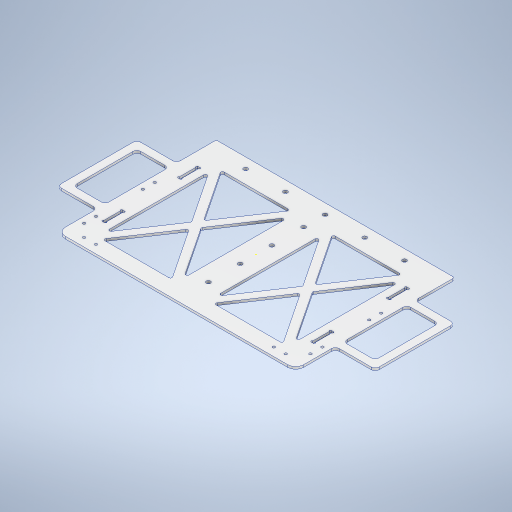
# Autodesk Inventor part: RP_Waist-Avobe-ver2
Saved by Autodesk Inventor 2024.3 (Build 283343000, 343)
## iProperties
Created: 2025-04-20
Part Number: RP_Waist-Avobe-ver2
Material: アルミニウム 6061
Document SubType Name: Modeling
Designer: ngt-a
Density: 2.7 g/cm^3
Appearance: アルミニウム - フラット
Mass: 310.216 g
Surface Area: 892.206 cm^2
Volume: 114.895 cm^3
Author: ngt-a
Autodesk Inventor part; units mm, degrees
ref_plane "YZ Plane" through (0, 0, 0) normal (1, 0, 0) x (0, 1, 0)
ref_plane "XZ Plane" through (0, 0, 0) normal (0, 1, 0) x (-1, 0, 0)
ref_plane "XY Plane" through (0, 0, 0) normal (0, 0, 1) x (1, 0, 0)
sketch "スケッチ1" plane through (0, 0, 0) normal (0, 1, 0) x (-1, 0, 0)
  line L0 (150, -95) -> (-150, -95)
  line L1 (-150, -95) -> (-150, 95)
  line L2 (-150, 95) -> (150, 95)
  line L3 (150, 95) -> (150, -95)
  line L4 (150, -95) -> (-150, 95) construction
  line L5 (-150, -95) -> (150, 95) construction
  line L6 (150, 95) -> (-150, 95)
  line L7 (-150, 95) -> (-150, 100)
  line L8 (-150, 100) -> (150, 100)
  line L9 (150, 100) -> (150, 95)
  line L10 (150, -50) -> (200, -50)
  line L11 (200, -50) -> (200, 50)
  line L12 (200, 50) -> (150, 50)
  line L13 (150, 50) -> (150, -50)
  line L14 (-150, -50) -> (-200, -50)
  line L15 (-200, -50) -> (-200, 50)
  line L16 (-200, 50) -> (-150, 50)
  line L17 (-150, 50) -> (-150, -50)
  line L18 (190, -40) -> (160, -40)
  line L19 (160, -40) -> (160, 40)
  line L20 (160, 40) -> (190, 40)
  line L21 (190, 40) -> (190, -40)
  line L22 (-190, -40) -> (-160, -40)
  line L23 (-160, -40) -> (-160, 40)
  line L24 (-160, 40) -> (-190, 40)
  line L25 (-190, 40) -> (-190, -40)
  line L26 (160, -40) -> (150, -40)
  line L27 (150, -40) -> (150, 40)
  line L28 (150, 40) -> (160, 40)
  line L29 (160, 40) -> (160, -40)
  line L30 (-160, -40) -> (-150, -40)
  line L31 (-150, -40) -> (-150, 40)
  line L32 (-150, 40) -> (-160, 40)
  line L33 (-160, 40) -> (-160, -40)
  point P0 (0, 0)
  point P1 (150, 0)
  point P2 (175, -40)
  point P3 (-155, -40)
  point P4 (-155, 40)
  point P5 (-150, 40)
  point P6 (150, 40)
  dimension "d0" = 190
  dimension "d1" = 300
  dimension "d244" = 5
  dimension "d346" = 50
  dimension "d347" = 50
  dimension "d348" = 50
  dimension "d349" = 50
  dimension "d350" = 10
  dimension "d351" = 10
  dimension "d352" = 80
  constraints: 68 end point, 16 parallel, 8 perpendicular, 6 horizontal, 6 midpoint, 6 point on line, 6 other
  measures "d0" distance of L0.end L1.end
  measures "d1" distance of L0.start L0.end
  measures "d244" distance between parallel lines of L2 L8
  measures "d346" distance between parallel lines of L13 L11
  measures "d347" distance from line of point (0, 0) L10
  measures "d348" distance from line of L12 point (150, 0)
  measures "d349" distance between parallel lines of L17 L15
  measures "d350" distance from line of L10 point (175, -40)
  measures "d351" distance between parallel lines of L14 L22
  measures "d352" distance of point (-155, -40) point (-155, 40)
extrude "押し出し1" add sketch "スケッチ1" along normal blind 3 contours L0 L1 L2 L3 | L3 L26 L18 L21 L20 L28 L12 L11 L10 | L14 L15 L16 L1 L32 L24 L25 L22 L30 | L2 L7 L8 L9
sketch "スケッチ2" plane through (0, 3, 0) normal (0, 1, 0) x (1, 0, 0)
  circle A0 centre (-142.5, -74) radius 1.6
  circle A1 centre (142.5, -74) radius 1.6
  line L0 (-150, -95) -> (150, -95) projected
  circle A2 centre (-142.5, -59) radius 1.6
  circle A3 centre (142.5, -59) radius 1.6
  circle A4 centre (-127, -89.5) radius 1.6
  line L1 (-150, 95) -> (-150, -100) projected
  circle A5 centre (-112, -89.5) radius 1.6
  line L2 (150, 95) -> (-150, 95) projected
  line L3 (0, 95) -> (0, -95)
  line L4 (-150, -2.5) -> (150, 0)
  line L5 (150, -95) -> (150, 95) projected
  circle A6 centre (127, -89.5) radius 1.6
  circle A7 centre (112, -89.5) radius 1.6
  circle A8 centre (-142.5, 15) radius 1.6
  circle A9 centre (-142.5, 0) radius 1.6
  circle A10 centre (142.5, 15) radius 1.6
  circle A11 centre (142.5, 0) radius 1.6
  point P0 (0, 0)
  dimension "d55" = 142.5
  dimension "d56" = 285
  dimension "d57" = 3.2
  dimension "d58" = 3.2
  dimension "d59" = 21
  dimension "d60" = 21
  dimension "d61" = 15
  dimension "d62" = 15
  dimension "d63" = 3.2
  dimension "d64" = 3.2
  dimension "d67" = 5.5
  dimension "d68" = 23
  dimension "d69" = 15
  dimension "d70" = 3.2
  dimension "d71" = 3.2
  dimension "d72" = 80
  dimension "d73" = 7.5
  dimension "d74" = 15
  dimension "d75" = 3.2
  dimension "d76" = 3.2
  dimension "d245" = 3.2
  constraints: 12 centre point, 4 end point, 4 midpoint, 4 symmetric about line, 4 other
  measures "d55" horizontal distance of A0.centre point (0, 0)
  measures "d56" distance of A1.centre A0.centre
  measures "d57" diameter of A0
  measures "d58" diameter of A1
  measures "d59" distance from line of L0 A0.centre
  measures "d60" distance from line of L0 A1.centre
  measures "d61" distance of A0.centre A2.centre
  measures "d62" distance of A1.centre A3.centre
  measures "d63" diameter of A3
  measures "d64" diameter of A2
  measures "d67" distance from line of L0 A4.centre
  measures "d68" distance from line of A4.centre L1
  measures "d69" distance of A5.centre A4.centre
  measures "d70" diameter of A5
  measures "d71" diameter of A4
  measures "d72" distance from line of A8.centre L2
  measures "d73" distance from line of A8.centre L1
  measures "d74" distance of A9.centre A8.centre
  measures "d75" diameter of A9
  measures "d76" diameter of A8
  measures "d245" diameter of A7
extrude "押し出し4" cut sketch "スケッチ2" against normal blind 10 contours A0 | A1 | A11 L4 | L4 A11 | A2 | A3 | A4 | A5 | A6 | A7 | A8 | A9 | A10
sketch "スケッチ4" plane through (0, 3, 0) normal (0, 1, 0) x (1, 0, 0)
  point P0 (0, 0)
sketch "スケッチ14" plane through (150, 0, -95) normal (0, 0, -1) x (-1, 0, 0)
  line L0 (0, 0) -> (300, 0) projected
  line L1 (300, 0) -> (300, 3) projected
  line L2 (0, 3) -> (300, 3) projected
  line L3 (0, 0) -> (0, 3) projected
  point P0 (150, 0)
extrude "押し出し13" add sketch "スケッチ14" along normal blind 5
fillet "フィレット3" radius 10 2 edges at (150, 1.5, 100) (-150, 1.5, 100)
sketch "スケッチ19" plane through (0, 0, 0) normal (0, -1, 0) x (1, 0, 0)
  circle A0 centre (-142.5, -15) radius 1.6 projected
  circle A1 centre (127, 89.5) radius 1.6 projected
  circle A2 centre (142.5, 74) radius 1.6 projected
  circle A3 centre (-142.5, 59) radius 1.6 projected
  circle A4 centre (-112, 89.5) radius 1.6 projected
  circle A5 centre (142.5, 0) radius 1.6 projected
  circle A6 centre (-142.5, 0) radius 1.6 projected
  circle A7 centre (112, 89.5) radius 1.6 projected
  circle A8 centre (142.5, 59) radius 1.6 projected
  circle A9 centre (-142.5, 74) radius 1.6 projected
  circle A10 centre (-127, 89.5) radius 1.6 projected
  circle A11 centre (142.5, -15) radius 1.6 projected
  line L0 (150, -40) -> (190, -40) projected
  line L1 (150, 40) -> (150, -40) projected
  line L2 (190, 40) -> (150, 40) projected
  line L3 (190, -40) -> (190, 40) projected
  line L4 (-150, 40) -> (-190, 40) projected
  line L5 (-150, -40) -> (-150, 40) projected
  line L6 (-190, -40) -> (-150, -40) projected
  line L7 (-190, 40) -> (-190, -40) projected
  arc A12 (-140, 100) -> (-150, 90) centre (-140, 90) ccw projected
  line L8 (-150, 50) -> (-150, 90) projected
  line L9 (-200, 50) -> (-150, 50) projected
  line L10 (-200, -50) -> (-200, 50) projected
  line L11 (-150, -50) -> (-200, -50) projected
  line L12 (-150, -50) -> (-150, -100) projected
  line L13 (150, -100) -> (-150, -100) projected
  line L14 (150, -50) -> (150, -100) projected
  line L15 (200, -50) -> (150, -50) projected
  line L16 (200, 50) -> (200, -50) projected
  line L17 (150, 50) -> (200, 50) projected
  line L18 (150, 90) -> (150, 50) projected
  arc A13 (150, 90) -> (140, 100) centre (140, 90) ccw projected
  line L19 (-140, 100) -> (140, 100) projected
  line L20 (120, -70) -> (20, -70)
  line L21 (20, -70) -> (20, 80)
  line L22 (20, 80) -> (120, 80)
  line L23 (120, 80) -> (120, -70)
  line L24 (-20, -70) -> (-120, -70)
  line L25 (-120, -70) -> (-120, 80)
  line L26 (-120, 80) -> (-20, 80)
  line L27 (-20, 80) -> (-20, -70)
  line L28 (150, -100) -> (-150, -100) projected
  line L29 (120, -70) -> (20, 80)
  line L30 (-20, 80) -> (-120, -70)
  line L31 (-20, -70) -> (-120, 80)
  line L32 (20, -70) -> (120, 80)
  line L33 (15.8397, -67.2265) -> (120.5004, 89.7644)
  line L34 (24.1603, -72.7735) -> (128.8209, 84.2174)
  line L35 (115.8397, -72.7735) -> (11.1791, 84.2174)
  line L36 (124.1603, -67.2265) -> (19.4996, 89.7644)
  line L37 (-15.8397, -67.2265) -> (-120.5004, 89.7644)
  line L38 (-24.1603, -72.7735) -> (-128.8209, 84.2174)
  line L39 (-19.4996, 89.7644) -> (-124.1603, -67.2265)
  line L40 (-11.1791, 84.2174) -> (-115.8397, -72.7735)
  point P0 (0, -100)
  point P1 (0, -100)
  point P2 (-70, 14.0139)
  point P3 (-26.0093, 80)
  point P4 (-113.9907, 80)
  point P5 (-120, -60.9861)
  point P6 (-76.0093, 5)
  point P7 (-120, 70.9861)
  point P8 (-70, -4.0139)
  point P9 (-113.9907, -70)
  point P10 (-26.0093, -70)
  point P11 (-20, 70.9861)
  point P12 (-63.9907, 5)
  point P13 (-20, -60.9861)
  point P14 (26.0093, 80)
  point P15 (70, 14.0139)
  point P16 (113.9907, 80)
  point P17 (63.9907, 5)
  point P18 (20, 70.9861)
  point P19 (20, -60.9861)
  point P20 (76.0093, 5)
  point P21 (120, -60.9861)
  point P22 (120, 70.9861)
  point P23 (113.9907, -70)
  point P24 (70, -4.0139)
  point P25 (26.0093, -70)
  dimension "d355" = 30
  dimension "d356" = 20
  dimension "d357" = 30
  dimension "d358" = 30
  dimension "d359" = 20
  dimension "d360" = 20
  dimension "d361" = 5
  dimension "d362" = 5
  dimension "d363" = 5
  dimension "d364" = 5
  dimension "d365" = 5
  dimension "d366" = 5
  dimension "d367" = 5
  dimension "d368" = 5
  constraints: 40 end point, 12 parallel, 2 horizontal, 2 midpoint, 2 perpendicular, 2 point on line
  measures "d355" distance between parallel lines of L13 L20
  measures "d356" distance between parallel lines of L19 L22
  measures "d357" distance between parallel lines of L1 L23
  measures "d358" distance between parallel lines of L5 L25
  measures "d359" distance from line of point (0, -100) L21
  measures "d360" distance from line of point (0, -100) L27
  measures "d361" distance between parallel lines of L35 L29
  measures "d362" distance between parallel lines of L36 L29
  measures "d363" distance between parallel lines of L32 L34
  measures "d364" distance between parallel lines of L33 L32
  measures "d365" distance between parallel lines of L31 L38
  measures "d366" distance between parallel lines of L37 L31
  measures "d367" distance between parallel lines of L40 L30
  measures "d368" distance between parallel lines of L39 L30
extrude "押し出し18" cut sketch "スケッチ19" against normal through all contours L20 L34 L35 | L36 L34 L23 | L21 L35 L33 | L33 L36 L22 | L24 L40 L38 | L37 L40 L27 | L25 L38 L39 | L39 L37 L26
sketch "スケッチ20" plane through (0, 0, 0) normal (0, -1, 0) x (1, 0, 0)
  line L0 (133, 35.4) -> (130, 35.4)
  line L1 (130, 35.4) -> (130, 60.4)
  line L2 (130, 60.4) -> (133, 60.4)
  line L3 (133, 60.4) -> (133, 35.4)
  circle A0 centre (127, 89.5) radius 1.6 projected
  line L4 (133, -59.6) -> (130, -59.6)
  line L5 (130, -59.6) -> (130, -34.6)
  line L6 (130, -34.6) -> (133, -34.6)
  line L7 (133, -34.6) -> (133, -59.6)
  arc A1 (133, -59.6) -> (133, -57.6) centre (133, -58.6) ccw
  arc A2 (130, -57.6) -> (130, -59.6) centre (130, -58.6) ccw
  arc A3 (133, -36.6) -> (133, -34.6) centre (133, -35.6) ccw
  arc A4 (130, -34.6) -> (130, -36.6) centre (130, -35.6) ccw
  arc A5 (133, 58.4) -> (133, 60.4) centre (133, 59.4) ccw
  arc A6 (130, 60.4) -> (130, 58.4) centre (130, 59.4) ccw
  arc A7 (133, 35.4) -> (133, 37.4) centre (133, 36.4) ccw
  arc A8 (130, 37.4) -> (130, 35.4) centre (130, 36.4) ccw
  line L8 (0, 0) -> (0, 29.3825)
  line L9 (-133, 35.4) -> (-130, 35.4)
  line L10 (-130, 35.4) -> (-130, 60.4)
  line L11 (-130, 60.4) -> (-133, 60.4)
  line L12 (-133, 60.4) -> (-133, 35.4)
  line L13 (-133, -59.6) -> (-130, -59.6)
  line L14 (-130, -59.6) -> (-130, -34.6)
  line L15 (-130, -34.6) -> (-133, -34.6)
  line L16 (-133, -34.6) -> (-133, -59.6)
  arc A9 (-133, -57.6) -> (-133, -59.6) centre (-133, -58.6) ccw
  arc A10 (-130, -59.6) -> (-130, -57.6) centre (-130, -58.6) ccw
  arc A11 (-133, -34.6) -> (-133, -36.6) centre (-133, -35.6) ccw
  arc A12 (-130, -36.6) -> (-130, -34.6) centre (-130, -35.6) ccw
  arc A13 (-133, 60.4) -> (-133, 58.4) centre (-133, 59.4) ccw
  arc A14 (-130, 58.4) -> (-130, 60.4) centre (-130, 59.4) ccw
  arc A15 (-133, 37.4) -> (-133, 35.4) centre (-133, 36.4) ccw
  arc A16 (-130, 35.4) -> (-130, 37.4) centre (-130, 36.4) ccw
  point P0 (131.5, 60.4)
  point P1 (131.5, 35.4)
  point P2 (131.5, -34.6)
  point P3 (-131.5, 60.4)
  point P4 (-131.5, 35.4)
  point P5 (-131.5, -34.6)
  dimension "d272" = 3
  dimension "d273" = 4.5
  dimension "d274" = 27.5
  dimension "d275" = 25
  dimension "d276" = 25
  dimension "d277" = 70
  dimension "d278" = 3
  dimension "d279" = 3
  dimension "d280" = 1
  dimension "d281" = 1
  dimension "d282" = 1
  dimension "d283" = 1
  dimension "d284" = 1
  dimension "d285" = 1
  dimension "d286" = 1
  dimension "d287" = 1
  constraints: 34 end point, 32 point on circle, 27 symmetric about line, 16 centre point, 16 point on line, 8 tangent, 4 parallel, 3 midpoint, 2 horizontal, 2 perpendicular, 1 vertical, 8 other
  measures "d272" distance between parallel lines of L1 L3
  measures "d273" horizontal distance of A0.centre point (131.5, 60.4)
  measures "d274" distance edge to line of A0 L2
  measures "d275" distance of point (131.5, 60.4) point (131.5, 35.4)
  measures "d276" distance of L6.end L4.start
  measures "d277" distance of point (131.5, 35.4) point (131.5, -34.6)
  measures "d278" distance between parallel lines of L5 L7
  measures "d279" distance from line of A0.centre L5
  measures "d280" radius of A1
  measures "d281" radius of A2
  measures "d282" radius of A3
  measures "d283" radius of A4
  measures "d284" radius of A5
  measures "d285" radius of A6
  measures "d286" radius of A7
  measures "d287" radius of A8
extrude "押し出し19" cut sketch "スケッチ20" against normal blind 5 contours L0 L1 L2 L3 | L3 A7 | A8 L1 | L3 A5 | A6 L1 | L4 L5 L6 L7 | L7 A1 | A2 L5 | L7 A3 | A4 L5 | L12 L11 L10 L9 | A15 L12 | L10 A16 | A13 L12 | L10 A14 | L16 L15 L14 L13 | A9 L16 | L14 A10 | A11 L16 | L14 A12
fillet "フィレット11" radius 2 24 edges at (26.0093, 1.5, -70) (-113.9907, 1.5, -70) (76.0093, 1.5, 5) (-63.9907, 1.5, 5) (63.9907, 1.5, 5) (113.9907, 1.5, -70) (-26.0093, 1.5, -70) (-20, 1.5, -60.9861) (-70, 1.5, 14.0139) (120, 1.5, -60.9861) (70, 1.5, 14.0139) (-76.0093, 1.5, 5) (70, 1.5, -4.0139) (-70, 1.5, -4.0139) (-20, 1.5, 70.9861) (120, 1.5, 70.9861) (26.0093, 1.5, 80) (-113.9907, 1.5, 80) (20, 1.5, 70.9861) (-120, 1.5, 70.9861) (-120, 1.5, -60.9861) (20, 1.5, -60.9861) (113.9907, 1.5, 80) (-26.0093, 1.5, 80)
fillet "フィレット12" radius 5 16 edges at (-200, 1.5, 50) (-200, 1.5, -50) (-150, 1.5, 50) (200, 1.5, 50) (150, 1.5, 50) (150, 1.5, -40) (200, 1.5, -50) (-150, 1.5, -40) (190, 1.5, -40) (190, 1.5, 40) (-150, 1.5, 40) (-190, 1.5, 40) (150, 1.5, 40) (-190, 1.5, -40) (150, 1.5, -50) (-150, 1.5, -50)
fillet "フィレット13" radius 2 2 edges at (150, 1.5, -100) (-150, 1.5, -100)
sketch "スケッチ21" plane through (0, 0, 0) normal (0, -1, 0) x (1, 0, 0)
  line L0 (-148, -100) -> (148, -100) projected
  line L1 (0, -100) -> (0, 100)
  line L2 (-140, 100) -> (140, 100) projected
  point P0 (0, 0)
  point P1 (0, -60)
  point P2 (0, -20)
  point P3 (0, 20)
  point P4 (0, 60)
  dimension "d369" = 40
  dimension "d370" = 40
  dimension "d371" = 40
  dimension "d372" = 40
  constraints: 4 point on line, 2 end point, 2 midpoint
  measures "d369" distance from line of L0 point (0, -60)
  measures "d370" distance of point (0, -60) point (0, -20)
  measures "d371" distance of point (0, -20) point (0, 20)
  measures "d372" distance of point (0, 20) point (0, 60)
hole "穴1" at (0, 0, -60) at (0, 0, -20) at (0, 0, 20) at (0, 0, 60) direction (0, 1, 0) diameter 5.2 end through all
sketch "スケッチ26" plane through (0, 3, 0) normal (0, 1, 0) x (1, 0, 0)
  line L0 (-150, 55) -> (-150, 98) projected
  line L1 (-150, 87) -> (150, 87)
  line L2 (-148, 100) -> (148, 100) projected
  line L3 (150, 55) -> (150, 98) projected
  point P0 (0, 0)
  point P1 (0, 87)
  point P2 (-50, 87)
  point P3 (-100, 87)
  point P4 (50, 87)
  point P5 (100, 87)
  point P6 (150, 76.5)
  dimension "d431" = 13
  dimension "d432" = 150
  dimension "d433" = 150
  dimension "d434" = 50
  dimension "d435" = 50
  dimension "d436" = 50
  dimension "d437" = 50
  constraints: 5 point on line, 2 end point, 2 midpoint, 1 horizontal
  measures "d431" distance between parallel lines of L2 L1
  measures "d432" horizontal distance of point (150, 76.5) point (0, 87)
  measures "d433" distance from line of L0 point (0, 87)
  measures "d434" distance of point (0, 87) point (-50, 87)
  measures "d435" distance of point (-50, 87) point (-100, 87)
  measures "d436" distance of point (0, 87) point (50, 87)
  measures "d437" distance of point (50, 87) point (100, 87)
hole "穴2" at (0, 3, -87) at (-50, 3, -87) at (-100, 3, -87) at (50, 3, -87) at (100, 3, -87) direction (0, -1, 0) diameter 5.2 end through all
sketch "スケッチ27" plane through (0, 3, 0) normal (0, 1, 0) x (1, 0, 0)
  circle A0 centre (100, 87) radius 2.6 projected
  circle A1 centre (50, 87) radius 2.6 projected
  circle A2 centre (-100, 87) radius 2.6 projected
  circle A3 centre (-50, 87) radius 2.6 projected
  circle A4 centre (0, 87) radius 2.6 projected
  circle A5 centre (0, -60) radius 2.6 projected
  circle A6 centre (0, -20) radius 2.6 projected
  circle A7 centre (0, 20) radius 2.6 projected
  circle A8 centre (0, 60) radius 2.6 projected
  arc A9 (-148, 100) -> (-150, 98) centre (-148, 98) ccw projected
  line L0 (-150, 55) -> (-150, 98) projected
  arc A10 (-155, 50) -> (-150, 55) centre (-155, 55) ccw projected
  line L1 (-155, 50) -> (-195, 50) projected
  arc A11 (-195, 50) -> (-200, 45) centre (-195, 45) ccw projected
  line L2 (-200, 45) -> (-200, -45) projected
  arc A12 (-200, -45) -> (-195, -50) centre (-195, -45) ccw projected
  line L3 (-195, -50) -> (-155, -50) projected
  arc A13 (-150, -55) -> (-155, -50) centre (-155, -55) ccw projected
  line L4 (-150, -55) -> (-150, -90) projected
  arc A14 (-150, -90) -> (-140, -100) centre (-140, -90) ccw projected
  line L5 (-140, -100) -> (140, -100) projected
  arc A15 (140, -100) -> (150, -90) centre (140, -90) ccw projected
  line L6 (150, -90) -> (150, -55) projected
  arc A16 (155, -50) -> (150, -55) centre (155, -55) ccw projected
  line L7 (155, -50) -> (195, -50) projected
  arc A17 (195, -50) -> (200, -45) centre (195, -45) ccw projected
  line L8 (200, -45) -> (200, 45) projected
  arc A18 (200, 45) -> (195, 50) centre (195, 45) ccw projected
  line L9 (195, 50) -> (155, 50) projected
  arc A19 (150, 55) -> (155, 50) centre (155, 55) ccw projected
  line L10 (150, 55) -> (150, 98) projected
  arc A20 (150, 98) -> (148, 100) centre (148, 98) ccw projected
  line L11 (-148, 100) -> (148, 100) projected
  line L12 (-133, 36.6) -> (-133, 57.6) projected
  arc A21 (-133, 59.6) -> (-133, 57.6) centre (-133, 58.6) ccw projected
  line L13 (-133, 59.6) -> (-130, 59.6) projected
  arc A22 (-130, 57.6) -> (-130, 59.6) centre (-130, 58.6) ccw projected
  line L14 (-130, 57.6) -> (-130, 36.6) projected
  arc A23 (-130, 34.6) -> (-130, 36.6) centre (-130, 35.6) ccw projected
  line L15 (-130, 34.6) -> (-133, 34.6) projected
  arc A24 (-133, 36.6) -> (-133, 34.6) centre (-133, 35.6) ccw projected
  arc A25 (133, -60.4) -> (133, -58.4) centre (133, -59.4) ccw projected
  line L16 (133, -60.4) -> (130, -60.4) projected
  arc A26 (130, -58.4) -> (130, -60.4) centre (130, -59.4) ccw projected
  line L17 (130, -58.4) -> (130, -37.4) projected
  arc A27 (130, -35.4) -> (130, -37.4) centre (130, -36.4) ccw projected
  line L18 (130, -35.4) -> (133, -35.4) projected
  arc A28 (133, -37.4) -> (133, -35.4) centre (133, -36.4) ccw projected
  line L19 (133, -37.4) -> (133, -58.4) projected
  arc A29 (-130, -60.4) -> (-130, -58.4) centre (-130, -59.4) ccw projected
  line L20 (-130, -60.4) -> (-133, -60.4) projected
  arc A30 (-133, -58.4) -> (-133, -60.4) centre (-133, -59.4) ccw projected
  line L21 (-133, -58.4) -> (-133, -37.4) projected
  arc A31 (-133, -35.4) -> (-133, -37.4) centre (-133, -36.4) ccw projected
  line L22 (-133, -35.4) -> (-130, -35.4) projected
  arc A32 (-130, -37.4) -> (-130, -35.4) centre (-130, -36.4) ccw projected
  line L23 (-130, -37.4) -> (-130, -58.4) projected
  line L24 (133, 57.6) -> (133, 36.6) projected
  arc A33 (133, 34.6) -> (133, 36.6) centre (133, 35.6) ccw projected
  line L25 (133, 34.6) -> (130, 34.6) projected
  arc A34 (130, 36.6) -> (130, 34.6) centre (130, 35.6) ccw projected
  line L26 (130, 36.6) -> (130, 57.6) projected
  arc A35 (130, 59.6) -> (130, 57.6) centre (130, 58.6) ccw projected
  line L27 (130, 59.6) -> (133, 59.6) projected
  arc A36 (133, 57.6) -> (133, 59.6) centre (133, 58.6) ccw projected
  line L28 (23.6641, 55.49) -> (63.2511, -3.8906) projected
  arc A37 (63.2511, -6.1094) -> (63.2511, -3.8906) centre (61.587, -5) ccw projected
  line L29 (63.2511, -6.1094) -> (23.6641, -65.49) projected
  arc A38 (20, -64.3806) -> (23.6641, -65.49) centre (22, -64.3806) ccw projected
  line L30 (20, -64.3806) -> (20, 54.3806) projected
  arc A39 (23.6641, 55.49) -> (20, 54.3806) centre (22, 54.3806) ccw projected
  line L31 (-120, -64.3806) -> (-120, 54.3806) projected
  arc A40 (-116.3359, 55.49) -> (-120, 54.3806) centre (-118, 54.3806) ccw projected
  line L32 (-116.3359, 55.49) -> (-76.7489, -3.8906) projected
  arc A41 (-76.7489, -6.1094) -> (-76.7489, -3.8906) centre (-78.413, -5) ccw projected
  line L33 (-76.7489, -6.1094) -> (-116.3359, -65.49) projected
  arc A42 (-120, -64.3806) -> (-116.3359, -65.49) centre (-118, -64.3806) ccw projected
  line L34 (-28.0822, 66.8906) -> (-68.3359, 6.51) projected
  arc A43 (-71.6641, 6.51) -> (-68.3359, 6.51) centre (-70, 7.6194) ccw projected
  line L35 (-71.6641, 6.51) -> (-111.9178, 66.8906) projected
  arc A44 (-110.2537, 70) -> (-111.9178, 66.8906) centre (-110.2537, 68) ccw projected
  line L36 (-110.2537, 70) -> (-29.7463, 70) projected
  arc A45 (-28.0822, 66.8906) -> (-29.7463, 70) centre (-29.7463, 68) ccw projected
  line L37 (116.3359, -65.49) -> (76.7489, -6.1094) projected
  arc A46 (76.7489, -3.8906) -> (76.7489, -6.1094) centre (78.413, -5) ccw projected
  line L38 (76.7489, -3.8906) -> (116.3359, 55.49) projected
  arc A47 (120, 54.3806) -> (116.3359, 55.49) centre (118, 54.3806) ccw projected
  line L39 (120, 54.3806) -> (120, -64.3806) projected
  arc A48 (116.3359, -65.49) -> (120, -64.3806) centre (118, -64.3806) ccw projected
  line L40 (110.2537, -80) -> (29.7463, -80) projected
  arc A49 (28.0822, -76.8906) -> (29.7463, -80) centre (29.7463, -78) ccw projected
  line L41 (28.0822, -76.8906) -> (68.3359, -16.51) projected
  arc A50 (71.6641, -16.51) -> (68.3359, -16.51) centre (70, -17.6194) ccw projected
  line L42 (71.6641, -16.51) -> (111.9178, -76.8906) projected
  arc A51 (110.2537, -80) -> (111.9178, -76.8906) centre (110.2537, -78) ccw projected
  line L43 (-111.9178, -76.8906) -> (-71.6641, -16.51) projected
  arc A52 (-68.3359, -16.51) -> (-71.6641, -16.51) centre (-70, -17.6194) ccw projected
  line L44 (-68.3359, -16.51) -> (-28.0822, -76.8906) projected
  arc A53 (-29.7463, -80) -> (-28.0822, -76.8906) centre (-29.7463, -78) ccw projected
  line L45 (-29.7463, -80) -> (-110.2537, -80) projected
  arc A54 (-111.9178, -76.8906) -> (-110.2537, -80) centre (-110.2537, -78) ccw projected
  line L46 (-20, 54.3806) -> (-20, -64.3806) projected
  arc A55 (-23.6641, -65.49) -> (-20, -64.3806) centre (-22, -64.3806) ccw projected
  line L47 (-23.6641, -65.49) -> (-63.2511, -6.1094) projected
  arc A56 (-63.2511, -3.8906) -> (-63.2511, -6.1094) centre (-61.587, -5) ccw projected
  line L48 (-63.2511, -3.8906) -> (-23.6641, 55.49) projected
  arc A57 (-20, 54.3806) -> (-23.6641, 55.49) centre (-22, 54.3806) ccw projected
  line L49 (29.7463, 70) -> (110.2537, 70) projected
  arc A58 (111.9178, 66.8906) -> (110.2537, 70) centre (110.2537, 68) ccw projected
  line L50 (111.9178, 66.8906) -> (71.6641, 6.51) projected
  arc A59 (68.3359, 6.51) -> (71.6641, 6.51) centre (70, 7.6194) ccw projected
  line L51 (68.3359, 6.51) -> (28.0822, 66.8906) projected
  arc A60 (29.7463, 70) -> (28.0822, 66.8906) centre (29.7463, 68) ccw projected
  circle A61 centre (-142.5, 15) radius 1.6 projected
  circle A62 centre (127, -89.5) radius 1.6 projected
  circle A63 centre (142.5, -74) radius 1.6 projected
  circle A64 centre (-142.5, -59) radius 1.6 projected
  circle A65 centre (-112, -89.5) radius 1.6 projected
  circle A66 centre (142.5, 0) radius 1.6 projected
  circle A67 centre (-142.5, 0) radius 1.6 projected
  circle A68 centre (112, -89.5) radius 1.6 projected
  circle A69 centre (142.5, -59) radius 1.6 projected
  circle A70 centre (-142.5, -74) radius 1.6 projected
  circle A71 centre (-127, -89.5) radius 1.6 projected
  circle A72 centre (142.5, 15) radius 1.6 projected
  line L52 (155, 40) -> (185, 40) projected
  arc A73 (190, 35) -> (185, 40) centre (185, 35) ccw projected
  line L53 (190, 35) -> (190, -35) projected
  arc A74 (185, -40) -> (190, -35) centre (185, -35) ccw projected
  line L54 (185, -40) -> (155, -40) projected
  arc A75 (150, -35) -> (155, -40) centre (155, -35) ccw projected
  line L55 (150, -35) -> (150, 35) projected
  arc A76 (155, 40) -> (150, 35) centre (155, 35) ccw projected
  line L56 (-155, -40) -> (-185, -40) projected
  arc A77 (-190, -35) -> (-185, -40) centre (-185, -35) ccw projected
  line L57 (-190, -35) -> (-190, 35) projected
  arc A78 (-185, 40) -> (-190, 35) centre (-185, 35) ccw projected
  line L58 (-185, 40) -> (-155, 40) projected
  arc A79 (-150, 35) -> (-155, 40) centre (-155, 35) ccw projected
  line L59 (-150, 35) -> (-150, -35) projected
  arc A80 (-155, -40) -> (-150, -35) centre (-155, -35) ccw projected
  line L60 (-130, 59.7) -> (-133, 59.7)
  arc A81 (-133, 59.7) -> (-133.1, 57.5046) centre (-133, 58.6) ccw
  line L61 (-133.1, 57.5046) -> (-133.1, 36.6954)
  arc A82 (-133.1, 36.6954) -> (-133, 34.5) centre (-133, 35.6) ccw
  line L62 (-133, 34.5) -> (-130, 34.5)
  arc A83 (-130, 34.5) -> (-129.9, 36.6954) centre (-130, 35.6) ccw
  line L63 (-129.9, 36.6954) -> (-129.9, 57.5046)
  arc A84 (-129.9, 57.5046) -> (-130, 59.7) centre (-130, 58.6) ccw
  line L64 (-130, -35.3) -> (-133, -35.3)
  arc A85 (-133, -35.3) -> (-133.1, -37.4954) centre (-133, -36.4) ccw
  line L65 (-133.1, -37.4954) -> (-133.1, -58.3046)
  arc A86 (-133.1, -58.3046) -> (-133, -60.5) centre (-133, -59.4) ccw
  line L66 (-133, -60.5) -> (-130, -60.5)
  arc A87 (-130, -60.5) -> (-129.9, -58.3046) centre (-130, -59.4) ccw
  line L67 (-129.9, -58.3046) -> (-129.9, -37.4954)
  arc A88 (-129.9, -37.4954) -> (-130, -35.3) centre (-130, -36.4) ccw
  line L68 (0, 100) -> (0, -100)
  line L69 (133, 36.6) -> (133, 57.6)
  arc A89 (133, 57.6) -> (133, 59.6) centre (133, 58.6) ccw
  line L70 (133, 59.6) -> (130, 59.6)
  arc A90 (130, 59.6) -> (130, 57.6) centre (130, 58.6) ccw
  line L71 (130, 57.6) -> (130, 36.6)
  arc A91 (130, 36.6) -> (130, 34.6) centre (130, 35.6) ccw
  line L72 (130, 34.6) -> (133, 34.6)
  arc A92 (133, 34.6) -> (133, 36.6) centre (133, 35.6) ccw
  arc A93 (130, -58.4) -> (130, -60.4) centre (130, -59.4) ccw
  line L73 (130, -60.4) -> (133, -60.4)
  arc A94 (133, -60.4) -> (133, -58.4) centre (133, -59.4) ccw
  line L74 (133, -58.4) -> (133, -37.4)
  arc A95 (133, -37.4) -> (133, -35.4) centre (133, -36.4) ccw
  line L75 (133, -35.4) -> (130, -35.4)
  arc A96 (130, -35.4) -> (130, -37.4) centre (130, -36.4) ccw
  line L76 (130, -37.4) -> (130, -58.4)
  line L77 (130, 59.7) -> (133, 59.7)
  arc A97 (133.1, 57.5046) -> (133, 59.7) centre (133, 58.6) ccw
  line L78 (133.1, 57.5046) -> (133.1, 36.6954)
  arc A98 (133, 34.5) -> (133.1, 36.6954) centre (133, 35.6) ccw
  line L79 (133, 34.5) -> (130, 34.5)
  arc A99 (129.9, 36.6954) -> (130, 34.5) centre (130, 35.6) ccw
  line L80 (129.9, 36.6954) -> (129.9, 57.5046)
  arc A100 (130, 59.7) -> (129.9, 57.5046) centre (130, 58.6) ccw
  line L81 (130, -35.3) -> (133, -35.3)
  arc A101 (133.1, -37.4954) -> (133, -35.3) centre (133, -36.4) ccw
  line L82 (133.1, -37.4954) -> (133.1, -58.3046)
  arc A102 (133, -60.5) -> (133.1, -58.3046) centre (133, -59.4) ccw
  line L83 (133, -60.5) -> (130, -60.5)
  arc A103 (129.9, -58.3046) -> (130, -60.5) centre (130, -59.4) ccw
  line L84 (129.9, -58.3046) -> (129.9, -37.4954)
  arc A104 (130, -35.3) -> (129.9, -37.4954) centre (130, -36.4) ccw
  point P0 (0, 0)
  dimension "d445" = 0.1
  dimension "d446" = 0.1
  constraints: 50 end point, 48 point on circle, 24 centre point, 24 symmetric about line, 2 midpoint, 30 other
  measures "d445" distance between parallel lines of L14 L63
  measures "d446" distance between parallel lines of L23 L67
extrude "押し出し22" cut sketch "スケッチ27" against normal through all contours A84 L63 A83 L62 A82 L61 A81 L60 | A88 L67 A87 L66 A86 L65 A85 L64 | L77 A97 L78 A98 L79 A99 L80 A100 | L81 A101 L82 A102 L83 A103 L84 A104
